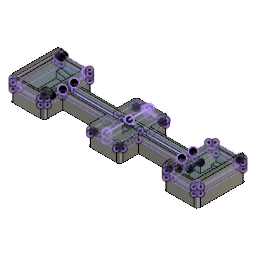
Sonaptic (Autodesk Fusion 360 design; units mm, degrees)
Autodesk Fusion 360 part; units mm, degrees
sketch "Bottom_Profile1" plane through (0, 0, 0) normal (0, 0, 1) x (1, 0, 0) in component "Bottom"
  line L0 (16, -30) -> (-16, -30)
  line L1 (-20, -26) -> (-20, 26)
  line L2 (-16, 30) -> (16, 30)
  line L3 (20, 26) -> (20, -26)
  line L4 (20, -30) -> (-20, 30) construction
  line L5 (-20, -30) -> (20, 30) construction
  line L6 (-11.5, 30) -> (11.5, 30)
  line L7 (11.5, 30) -> (11.5, -24)
  line L8 (11.5, -24) -> (-11.5, -24)
  line L9 (-11.5, -24) -> (-11.5, 30)
  line L10 (0, -24) -> (0, 30) construction
  line L11 (-11.5, 28) -> (11.5, 28)
  arc A0 (-16, 30) -> (-20, 26) centre (-16, 26) ccw
  arc A1 (20, 26) -> (16, 30) centre (16, 26) ccw
  arc A2 (16, -30) -> (20, -26) centre (16, -26) ccw
  arc A3 (-20, -26) -> (-16, -30) centre (-16, -26) ccw
  circle A4 centre (-16, 26) radius 1.25
  circle A5 centre (16, 26) radius 1.25
  circle A6 centre (16, -26) radius 1.25
  circle A7 centre (-16, -26) radius 1.25
  line L12 (0, 0) -> (75, 0) construction
  line L13 (111, -30) -> (77, -30)
  line L14 (73, -26) -> (73, 26)
  line L15 (77, 30) -> (111, 30)
  line L16 (115, 26) -> (115, -26)
  line L17 (115, -30) -> (73, 30) construction
  line L18 (73, -30) -> (115, 30) construction
  arc A8 (77, 30) -> (73, 26) centre (77, 26) ccw
  arc A9 (115, 26) -> (111, 30) centre (111, 26) ccw
  arc A10 (111, -30) -> (115, -26) centre (111, -26) ccw
  arc A11 (73, -26) -> (77, -30) centre (77, -26) ccw
  line L19 (20, 7) -> (73, 7)
  line L20 (20, -7) -> (73, -7)
  line L21 (-73, -30) -> (-115, 30) construction
  line L22 (-73, -26) -> (-73, 26)
  line L23 (-111, -30) -> (-77, -30)
  line L24 (-115, 26) -> (-115, -26)
  arc A12 (-111, 30) -> (-115, 26) centre (-111, 26) ccw
  line L25 (-115, -30) -> (-73, 30) construction
  arc A13 (-73, 26) -> (-77, 30) centre (-77, 26) ccw
  arc A14 (-77, -30) -> (-73, -26) centre (-77, -26) ccw
  arc A15 (-115, -26) -> (-111, -30) centre (-111, -26) ccw
  line L26 (-77, 30) -> (-111, 30)
  line L27 (-20, -7) -> (-73, -7)
  line L28 (-20, 7) -> (-73, 7)
  line L29 (0, 0) -> (-75, 0) construction
  circle A16 centre (-16, 26) radius 2
  circle A17 centre (16, 26) radius 2
  circle A18 centre (16, -26) radius 2
  circle A19 centre (-16, -26) radius 2
  line L30 (-73, 3.5) -> (73, 3.5)
  line L31 (73, 3.5) -> (73, -3.5)
  line L32 (73, -3.5) -> (-73, -3.5)
  line L33 (-73, -3.5) -> (-73, 3.5)
  line L34 (108, -26) -> (82, -26)
  line L35 (82, -26) -> (82, 26)
  line L36 (82, 26) -> (108, 26)
  line L37 (108, 26) -> (108, -26)
  line L38 (108, -26) -> (82, 26) construction
  line L39 (82, -26) -> (108, 26) construction
  line L40 (-82, 26) -> (-108, 26)
  line L41 (-82, -26) -> (-82, 26)
  line L42 (-108, -26) -> (-82, 26) construction
  line L43 (-82, -26) -> (-108, 26) construction
  line L44 (-108, 26) -> (-108, -26)
  line L45 (-108, -26) -> (-82, -26)
  line L46 (73, 3.5) -> (82, 3.5)
  line L47 (73, -3.5) -> (82, -3.5)
  line L48 (-73, 3.5) -> (-82, 3.5)
  line L49 (-73, -3.5) -> (-82, -3.5)
  line L50 (82, 7) -> (75, 7)
  line L51 (82, -7) -> (75, -7)
  line L52 (75, 7) -> (75, -7)
  line L53 (-82, 7) -> (-75, 7)
  line L54 (-75, 7) -> (-75, -7)
  line L55 (-82, -7) -> (-75, -7)
  line L56 (82, -20) -> (108, -20)
  line L57 (95, 0) -> (108, 0) construction
  line L58 (82, 20) -> (108, 20)
  line L59 (-82, 20) -> (-108, 20)
  line L60 (-82, -20) -> (-108, -20)
  circle A20 centre (-5.75, 26) radius 1.25
  circle A21 centre (5.75, 26) radius 1.25
  circle A22 centre (-5.75, -21) radius 1.25
  circle A23 centre (5.75, -21) radius 1.25
  circle A24 centre (-5.75, 26) radius 2
  circle A25 centre (5.75, 26) radius 2
  circle A26 centre (-5.75, -21) radius 2
  circle A27 centre (5.75, -21) radius 2
  circle A28 centre (111, 26) radius 1.25
  circle A29 centre (111, 26) radius 2
  circle A30 centre (77, -26) radius 2
  circle A31 centre (77, -26) radius 1.25
  circle A32 centre (-111, 26) radius 1.25
  circle A33 centre (-111, 26) radius 2
  circle A34 centre (-77, -26) radius 2
  circle A35 centre (-77, -26) radius 1.25
  point P0 (92.9265, 0)
  point P1 (-92.9265, 0)
  point P2 (92.9265, 0)
  point P3 (95, 0)
  point P4 (94, 0)
  point P5 (95, -23)
  point P6 (95, 23)
  point P7 (-95, 23)
  point P8 (-95, -23)
  dimension "d1" = 40
  dimension "d2" = 60
  dimension "d3" = 23
  dimension "d4" = 54
  dimension "d5" = 2
  dimension "d6" = 4
  dimension "d7" = 2.5
  dimension "d8" = 75
  dimension "d9" = 42
  dimension "d10" = 4
  dimension "d11" = 60
  dimension "d12" = 14
  dimension "d15" = 4
  dimension "d16" = 7
  dimension "d17" = 26
  dimension "d18" = 52
  dimension "d19" = 2
  dimension "d22" = 9
  dimension "d23" = 7
  dimension "d24" = 14
  dimension "d29" = 3
  dimension "d30" = 3
  dimension "d31" = 11.5
  dimension "d32" = 2.5
  dimension "d36" = 2
  dimension "d37" = 11.5
  dimension "d38" = 3
  dimension "d39" = 4
  dimension "d46" = 2.5
  dimension "d47" = 4
  constraint horizontal L0
  constraint perpendicular L0 L1
  constraint parallel L0 L2
  constraint parallel L1 L3
  constraint coincident L4 L12.start
  constraint coincident L5 L12.start
  constraint coincident L12.start L29.start
  constraint horizontal L6
  constraint vertical L7
  constraint horizontal L8
  constraint vertical L9
  constraint coincident L2 L6.start
  constraint midpoint L8 L10.start
  constraint midpoint L6 L10.end
  constraint coincident L12.start L10
  constraint coincident L9 L11.start
  constraint coincident L7 L11.end
  constraint perpendicular L7 L11
  constraint coincident L4.end L1
  constraint coincident L4.end L2
  constraint tangent L1 A0
  constraint tangent L2 A0
  constraint coincident L5.end L2
  constraint coincident L5.end L3
  constraint tangent L2 A1
  constraint tangent L3 A1
  constraint equal A0 A1
  constraint coincident L4.start L3
  constraint coincident L4.start L0
  constraint tangent L3 A2
  constraint tangent L0 A2
  constraint equal A0 A2
  constraint coincident L5.start L0
  constraint coincident L5.start L1
  constraint tangent L0 A3
  constraint tangent L1 A3
  constraint equal A0 A3
  constraint concentric A0 A4
  constraint concentric A1 A5
  constraint equal A4 A5
  constraint concentric A2 A6
  constraint concentric A3 A7
  constraint equal A4 A6
  constraint equal A4 A7
  constraint perpendicular L10 L12
  constraint horizontal L13
  constraint perpendicular L13 L14
  constraint parallel L13 L15
  constraint parallel L14 L16
  constraint horizontal L12.end P2
  constraint coincident L17.end L14
  constraint coincident L17.end L15
  constraint tangent L14 A8
  constraint tangent L15 A8
  constraint coincident L18.end L15
  constraint coincident L18.end L16
  constraint tangent L15 A9
  constraint tangent L16 A9
  constraint equal A8 A9
  constraint coincident L17.start L16
  constraint coincident L17.start L13
  constraint tangent L16 A10
  constraint tangent L13 A10
  constraint equal A8 A10
  constraint coincident L18.start L13
  constraint coincident L18.start L14
  constraint tangent L13 A11
  constraint tangent L14 A11
  constraint equal A8 A11
  constraint coincident L3 L19.start
  constraint coincident L14 L19.end
  constraint perpendicular L14 L19
  constraint symmetric L12 L19.start L20.start
  constraint symmetric L12 L19.end L20.end
  constraint symmetric L10 L12.start L29.start
  constraint symmetric L10 L12.end L29.end
  constraint symmetric L10 L17.start L25.start
  constraint symmetric L10 L18.start L21.start
  constraint symmetric L10 L17.end L25.end
  constraint symmetric L10 L18.end L21.end
  constraint symmetric L10 P2 P1
  constraint symmetric L10 L14.end L22.end
  constraint symmetric L10 L15.start A13.end
  constraint symmetric L10 A8 A13
  constraint symmetric L10 L15.end A12.start
  constraint symmetric L10 L16.start L24.start
  constraint symmetric L10 A9 A12
  constraint symmetric L10 L16.end L24.end
  constraint symmetric L10 L13.start L23.start
  constraint symmetric L10 A10 A15
  constraint symmetric L10 L13.end L23.end
  constraint symmetric L10 L14.start L22.start
  constraint symmetric L10 A11 A14
  constraint symmetric L10 L19.start L28.start
  constraint symmetric L10 L19.end L28.end
  constraint symmetric L10 L20.start L27.start
  constraint symmetric L10 L20.end L27.end
  constraint concentric A0 A16
  constraint concentric A5 A17
  constraint concentric A6 A18
  constraint concentric A7 A19
  constraint equal A16 A17
  constraint equal A16 A18
  constraint equal A16 A19
  constraint horizontal L30
  constraint vertical L31
  constraint horizontal L32
  constraint vertical L33
  constraint coincident L14 L31.end
  constraint coincident L22 L30.start
  constraint symmetric L12 L30 L32
  constraint horizontal L34
  constraint perpendicular L34 L35
  constraint parallel L34 L36
  constraint parallel L35 L37
  constraint coincident P2 P0
  constraint symmetric L10 L34.start L42.start
  constraint symmetric L10 L34.end L41.start
  constraint symmetric L10 L35.end L40.start
  constraint symmetric L10 L36.end L40.end
  constraint coincident L35 L46.end
  constraint perpendicular L35 L46
  constraint coincident L35 L47.end
  constraint perpendicular L35 L47
  constraint symmetric L10 L30.end L30.start
  constraint symmetric L10 L31.end L32.end
  constraint symmetric L10 L46.end L48.end
  constraint symmetric L10 L47.end L49.end
  constraint midpoint L38 P3
  constraint horizontal P2 P3
  constraint coincident L35 L50.start
  constraint perpendicular L35 L50
  constraint symmetric L12 L50.start L51.start
  constraint symmetric L12 L50.end L51.end
  constraint symmetric L10 L50.start L53.start
  constraint symmetric L10 L50.end L53.end
  constraint symmetric L10 L51.start L55.start
  constraint symmetric L10 L51.end L54.end
  constraint midpoint L17 P4
  constraint horizontal P2 P4
  constraint coincident L35 L56.start
  constraint coincident L37 L56.end
  constraint perpendicular L37 L56
  constraint coincident P3 L57.start
  constraint midpoint L37 L57.end
  constraint symmetric P5 L57 P6
  constraint symmetric L56.start L57 L58.start
  constraint symmetric L56.end L57 L58.end
  constraint symmetric L10 P5 P8
  constraint symmetric L10 L56.start L60.start
  constraint symmetric L10 L56.end L60.end
  constraint symmetric L10 P6 P7
  constraint symmetric L10 L58.start L59.start
  constraint symmetric L10 L58.end L59.end
  constraint symmetric L10 A20 A21
  constraint symmetric L10 A22 A23
  constraint equal A20 A22
  constraint concentric A20 A24
  constraint symmetric L10 A24 A25
  constraint concentric A22 A26
  constraint equal A24 A26
  constraint symmetric L10 A26 A27
  constraint concentric A9 A28
  constraint concentric A9 A29
  constraint concentric A11 A30
  constraint concentric A11 A31
  constraint equal A28 A31
  constraint equal A29 A30
  constraint symmetric L10 A28 A32
  constraint symmetric L10 A29 A33
  constraint symmetric L10 A30 A34
  constraint symmetric L10 A31 A35
  measures "d1" distance of L4.end L5.end
  measures "d2" distance of L5.start L4.end
  measures "d3" distance of L6.start L6.end
  measures "d4" distance of L6.start L8.end
  measures "d5" distance of L6 L11
  measures "d6" radius of A0
  measures "d7" diameter of A4
  measures "d8" distance of L12.start L12.end
  measures "d9" distance of L17.end L18.end
  measures "d10" radius of A8
  measures "d11" distance of L13 L15
  measures "d12" distance of L19 L20
  measures "d15" diameter of A16
  measures "d16" distance of L30 L32
  measures "d17" distance of L35.end L36.end
  measures "d18" distance of L34.end L35.end
  measures "d19" distance of L12.end L14
  measures "d22" distance of L14 L35
  measures "d23" distance of L50.start L50.end
  measures "d24" distance of L50 L51
  measures "d29" distance of L34 P5
  measures "d30" distance of P5 L56
  measures "d31" distance of A20.centre A21.centre
  measures "d32" diameter of A20
  measures "d36" distance of L11 A20.centre
  measures "d37" distance of A22.centre A23.centre
  measures "d38" distance of L8 A23.centre
  measures "d39" diameter of A24
  measures "d46" diameter of A28
  measures "d47" diameter of A29
extrude "Extrude2" add sketch "Bottom_Profile1" along normal blind 15 contours L0 L1 L3 L7 L8 L9 A2 A3 L32 | L3 L14 L20 L32 | L1 L22 L27 L32 | L13 L14 L15 L16 A8 A9 A10 A11 L34 L35 L36 L37 L46 L47 L50 L51 L52 | L22 L23 L24 A12 A13 A14 A15 L26 L40 L41 L44 L45 L48 L49 L53 L54 L55 | L2 L3 L7 A1 L30 | L3 L14 L19 L30 | L1 L22 L28 L30 | L1 L2 L9 A0 L30 | A16 | A17 | A18 | A19 | A29 | A30 | A33 | A34 makes body 1 in component "Bottom"
extrude "Extrude3" add sketch "Bottom_Profile1" along normal blind 3 contours L3 L7 L30 L32 | L3 L14 L30 L31 L32 | L1 L22 L30 L32 L33 | L1 L9 L30 L32 | L14 L31 L46 L47 L52 | L7 L9 L30 L32 | L22 L33 L48 L49 L54 | L35 L46 L47 L52 | L35 L47 L51 L52 | L41 L49 L54 L55 | L41 L48 L49 L54 | L35 L46 L50 L52 | L35 L37 L56 L58 | L41 L48 L53 L54 | L41 L44 L59 L60 bodies 1 in component "Bottom"
extrude "Extrude4" add sketch "Bottom_Profile1" along normal blind 5 contours L7 L8 L9 L32 | A25 | A24 | L7 L9 L11 L30 | A26 | A27 bodies 1 in component "Bottom"
extrude "Extrude5" add sketch "Bottom_Profile1" along normal up to surface (6 mm away) contours L2 L6 L7 L9 L11 bodies 1 in component "Bottom"
extrude "Extrude6" add sketch "Bottom_Profile1" along normal blind 16 contours L34 L35 L37 L56 | L41 L44 L45 L60 | L35 L36 L37 L58 | L40 L41 L44 L59 bodies 1 in component "Bottom"
sketch "Slice_Profile1" plane through (0, 0, 0) normal (0, 1, 0) x (1, 0, 0) in component "Bottom"
  line L0 (82, -3) -> (82, -6) construction
  line L1 (82, -6) -> (82, -16)
  line L2 (108, -3) -> (108, -16) construction
  line L3 (82, -6) -> (108, -6) construction
  line L4 (82, -6) -> (108, -10.5845)
  line L5 (108, -10.5845) -> (108, -16)
  line L6 (108, -16) -> (82, -16)
  line L7 (0, -1.75) -> (0, -22.5)
  line L8 (-108, -16) -> (-82, -16)
  line L9 (-82, -6) -> (-108, -10.5845)
  line L10 (-82, -6) -> (-82, -16)
  line L11 (-108, -10.5845) -> (-108, -16)
  point P0 (108, -3)
  point P1 (82, -3)
  point P2 (108, -16)
  dimension "d48" = 3
  dimension "d49" = 10
  constraint coincident P1 L0.start
  constraint vertical L0
  constraint parallel L0 L1
  constraint coincident P0 L2.start
  constraint coincident P2 L2.end
  constraint coincident L2 L3.end
  constraint perpendicular L2 L3
  constraint coincident L2 L4.end
  constraint perpendicular L1 L6
  constraint symmetric L0.end L7 L9.start
  constraint symmetric L1.end L7 L8.end
  constraint symmetric L4.end L7 L9.end
  constraint symmetric P2 L7 L8.start
  measures "d48" distance of P1 L0.end
  measures "d49" angle of L3 L4
extrude "Extrude7" cut sketch "Slice_Profile1" along normal up to surface (26 mm away) and the other way up to surface (26 mm away) bodies 1 in component "Bottom"
sketch "Fastener_Profile1" plane through (-1.4465, 0, -8.2037) normal (0.173648, 0, 0.984808) x (0, 1, 0) in component "Bottom"
  line L0 (-20, 81.7961) -> (-20, 108.1972)
  line L1 (-20, 108.1972) -> (-26, 108.1972)
  line L2 (-26, 108.1972) -> (-26, 81.7961)
  line L3 (-26, 81.7961) -> (-20, 81.7961)
  circle A0 centre (-23, 94.9967) radius 2.25
  circle A1 centre (-23, 94.9967) radius 2
  circle A2 centre (-23, 94.9967) radius 1.25
  line L4 (-23, 108.1972) -> (-23, 81.7961) construction
  line L5 (-20, 94.9967) -> (-26, 94.9967) construction
  point P0 (-23, 93.5567)
  point P1 (-23, 94.9967)
  dimension "d55" = 4.5
  dimension "d56" = 4
  dimension "d57" = 2.5
  constraint midpoint L1 L4.start
  constraint midpoint L3 L4.end
  constraint coincident P1 L4
  constraint coincident P1 A0.centre
  constraint midpoint L0 L5.start
  constraint midpoint L2 L5.end
  constraint coincident L4 P1
  constraint coincident L5 P1
  measures "d55" diameter of A0
  measures "d56" diameter of A1
  measures "d57" diameter of A2
sketch "Fastener_Profile2" plane through (1.4465, 0, -8.2037) normal (-0.173648, 0, 0.984808) x (0, -1, 0) in component "Bottom"
  line L0 (-20, 81.7961) -> (-20, 108.1972)
  line L1 (-20, 108.1972) -> (-26, 108.1972)
  line L2 (-26, 108.1972) -> (-26, 81.7961)
  line L3 (-26, 81.7961) -> (-20, 81.7961)
  circle A0 centre (-23, 94.9967) radius 2.25
  circle A1 centre (-23, 94.9967) radius 2
  circle A2 centre (-23, 94.9967) radius 1.25
  line L4 (-23, 108.1972) -> (-23, 81.7961) construction
  line L5 (-26, 94.9967) -> (-20, 94.9967) construction
  point P0 (-23, 93.5567)
  point P1 (-23, 94.9967)
  dimension "d58" = 4.5
  dimension "d59" = 4
  dimension "d60" = 2.5
  constraint midpoint L1 L4.start
  constraint midpoint L3 L4.end
  constraint midpoint L2 L5.start
  constraint midpoint L0 L5.end
  constraint coincident L4 P1
  constraint coincident L5 P1
  constraint coincident P1 A0.centre
  measures "d58" diameter of A0
  measures "d59" diameter of A1
  measures "d60" diameter of A2
extrude "Extrude8" cut sketch "Fastener_Profile2" against normal blind 6 contours A2 bodies 1 in component "Bottom"
extrude "Extrude9" cut sketch "Fastener_Profile2" against normal blind 5 contours A1 bodies 1 in component "Bottom"
extrude "Extrude10" cut sketch "Fastener_Profile2" against normal blind 1 contours A0 bodies 1 in component "Bottom"
extrude "Extrude11" cut sketch "Fastener_Profile1" against normal blind 6 contours A2 bodies 1 in component "Bottom"
extrude "Extrude12" cut sketch "Fastener_Profile1" against normal blind 5 contours A1 bodies 1 in component "Bottom"
extrude "Extrude13" cut sketch "Fastener_Profile1" against normal blind 1 contours A0 bodies 1 in component "Bottom"
extrude "Extrude14" cut sketch "Bottom_Profile1" along normal blind 5 contours A16 | A17 | A18 | A19 | A29 | A30 | A33 | A34 bodies 1 in component "Bottom"
extrude "Extrude15" cut sketch "Bottom_Profile1" along normal blind 3 contours A25 | A24 | A26 | A27 bodies 1 in component "Bottom"
sketch "Top_Profile" plane through (0, 0, 15) normal (0, 0, 1) x (-1, 0, 0) in component "Top"
  circle A0 centre (111, -26) radius 1.25
  circle A1 centre (77, 26) radius 1.25
  circle A2 centre (-111, -26) radius 1.25
  circle A3 centre (16, 26) radius 1.25
  circle A4 centre (-16, 26) radius 1.25
  circle A5 centre (16, -26) radius 1.25
  circle A6 centre (-77, 26) radius 1.25
  circle A7 centre (-16, -26) radius 1.25
  line L0 (82, -7) -> (75, -7)
  line L1 (75, -7) -> (75, -3.5)
  line L2 (75, -3.5) -> (11.5, -3.5)
  line L3 (11.5, -3.5) -> (11.5, -30)
  line L4 (11.5, -30) -> (16, -30)
  arc A8 (16, -30) -> (20, -26) centre (16, -26) ccw
  line L5 (20, -26) -> (20, -7)
  line L6 (20, -7) -> (73, -7)
  line L7 (73, -7) -> (73, -26)
  arc A9 (73, -26) -> (77, -30) centre (77, -26) ccw
  line L8 (77, -30) -> (111, -30)
  arc A10 (111, -30) -> (115, -26) centre (111, -26) ccw
  line L9 (115, -26) -> (115, 26)
  arc A11 (115, 26) -> (111, 30) centre (111, 26) ccw
  line L10 (111, 30) -> (77, 30)
  arc A12 (77, 30) -> (73, 26) centre (77, 26) ccw
  line L11 (73, 26) -> (73, 7)
  line L12 (73, 7) -> (20, 7)
  line L13 (20, 7) -> (20, 26)
  arc A13 (20, 26) -> (16, 30) centre (16, 26) ccw
  line L14 (16, 30) -> (-16, 30)
  arc A14 (-16, 30) -> (-20, 26) centre (-16, 26) ccw
  line L15 (-20, 26) -> (-20, 7)
  line L16 (-20, 7) -> (-73, 7)
  line L17 (-73, 7) -> (-73, 26)
  arc A15 (-73, 26) -> (-77, 30) centre (-77, 26) ccw
  line L18 (-77, 30) -> (-111, 30)
  arc A16 (-111, 30) -> (-115, 26) centre (-111, 26) ccw
  line L19 (-115, 26) -> (-115, -26)
  arc A17 (-115, -26) -> (-111, -30) centre (-111, -26) ccw
  line L20 (-111, -30) -> (-77, -30)
  arc A18 (-77, -30) -> (-73, -26) centre (-77, -26) ccw
  line L21 (-73, -26) -> (-73, -7)
  line L22 (-73, -7) -> (-20, -7)
  line L23 (-20, -7) -> (-20, -26)
  arc A19 (-20, -26) -> (-16, -30) centre (-16, -26) ccw
  line L24 (-16, -30) -> (-11.5, -30)
  line L25 (-11.5, -30) -> (-11.5, -3.5)
  line L26 (-11.5, -3.5) -> (-75, -3.5)
  line L27 (-75, -3.5) -> (-75, -7)
  line L28 (-75, -7) -> (-82, -7)
  line L29 (-82, -7) -> (-82, -26)
  line L30 (-82, -26) -> (-108, -26)
  line L31 (-108, -26) -> (-108, 26)
  line L32 (-108, 26) -> (-82, 26)
  line L33 (-82, 26) -> (-82, 7)
  line L34 (-82, 7) -> (-75, 7)
  line L35 (-75, 7) -> (-75, 3.5)
  line L36 (-75, 3.5) -> (-11.5, 3.5)
  line L37 (-11.5, 3.5) -> (-11.5, 24)
  line L38 (-11.5, 24) -> (11.5, 24)
  line L39 (11.5, 24) -> (11.5, 3.5)
  line L40 (11.5, 3.5) -> (75, 3.5)
  line L41 (75, 3.5) -> (75, 7)
  line L42 (75, 7) -> (82, 7)
  line L43 (82, 7) -> (82, 26)
  line L44 (82, 26) -> (108, 26)
  line L45 (108, 26) -> (108, -26)
  line L46 (108, -26) -> (82, -26)
  line L47 (82, -26) -> (82, -7)
  line L48 (16, -30) -> (-16, -30)
  line L49 (11.5, -28) -> (-11.5, -28)
  line L50 (-11.5, -30) -> (11.5, -30)
  line L51 (11.5, -30) -> (11.5, -28)
  line L52 (11.5, -28) -> (-11.5, -28)
  line L53 (-11.5, -28) -> (-11.5, -30)
  circle A20 centre (16, 26) radius 2
  circle A21 centre (16, 26) radius 2.25
  circle A22 centre (-16, 26) radius 2
  circle A23 centre (-16, 26) radius 2.25
  circle A24 centre (-16, -26) radius 2
  circle A25 centre (16, -26) radius 2
  circle A26 centre (16, -26) radius 2.25
  circle A27 centre (-16, -26) radius 2.25
  line L54 (-82, 7) -> (-82, -7)
  line L55 (82, 7) -> (82, -7)
  dimension "d87" = 4
  dimension "d88" = 4.5
  constraint concentric A3 A20
  constraint concentric A3 A21
  constraint concentric A4 A22
  constraint concentric A22 A23
  constraint concentric A7 A24
  constraint concentric A5 A25
  constraint concentric A25 A26
  constraint concentric A24 A27
  constraint equal A21 A27
  constraint equal A21 A23
  constraint equal A21 A26
  constraint equal A20 A25
  constraint equal A20 A24
  constraint equal A20 A22
  constraint coincident L33.end L34.start
  constraint coincident L28.end L29.start
  constraint coincident L42.end L43.start
  constraint coincident L0.start L47.end
  measures "d87" diameter of A20
  measures "d88" diameter of A21
extrude "Extrude1" add sketch "Top_Profile" along normal blind 7 separate body contours A3 | A4 | A5 | A7 | L0 L1 L2 L3 L4 A8 L5 L6 L7 A9 L8 A10 L9 A11 L10 A12 L11 L12 L13 A13 L14 A14 L15 L16 L17 A15 L18 A16 L19 A17 L20 A18 L21 L22 L23 A19 L24 L25 L26 L27 L28 L29 L30 L31 L32 L33 L34 L35 L36 L37 L38 L39 L40 L41 L42 L43 L44 L45 L46 L47 L48 L51 L53 | L0 L1 L2 L3 L25 L26 L27 L28 L34 L35 L36 L37 L38 L39 L40 L41 L42 L49 L52 L54 L55 | L3 L25 L48 L49 L50 L51 L52 L53 | A20 | A21 | A22 | A23 | A24 | A25 | A26 | A27 makes body 2 in component "Top"
extrude "Extrude2'" add sketch "Top_Profile" against normal blind 3 contours L3 L25 L48 L49 L50 L51 L52 L53 bodies 2 in component "Top"
extrude "Extrude4'" cut sketch "Top_Profile" along normal blind 3 contours L43 L44 L45 L46 L47 L55 | L0 L1 L2 L3 L25 L26 L27 L28 L34 L35 L36 L37 L38 L39 L40 L41 L42 L49 L52 L54 L55 | L29 L30 L31 L32 L33 L54 bodies 2 in component "Top"
extrude "Extrude5'" cut sketch "Top_Profile" along normal blind 6 contours A3 | A4 | A5 | A7 bodies 2 in component "Top"
extrude "Extrude6'" cut sketch "Top_Profile" along normal blind 5 contours A20 | A22 | A24 | A25 bodies 2 in component "Top"
extrude "Extrude7'" cut sketch "Top_Profile" along normal blind 1 contours A21 | A23 | A26 | A27 bodies 2 in component "Top"
sketch "Side_Profile" plane through (0, 0, 0) normal (1, 0, 0) x (0, 1, 0) in component "Strip"
  line L0 (-26, 15) -> (26, 15)
  line L1 (-26, 22) -> (26, 22)
  circle A0 centre (0, 17.75) radius 6.25
  line L2 (6.25, 11.5) -> (-6.25, 11.5) construction
  line L3 (-6.25, 11.5) -> (-6.25, 24)
  line L4 (-6.25, 24) -> (6.25, 24) construction
  line L5 (6.25, 24) -> (6.25, 11.5)
  line L6 (6.25, 11.5) -> (-6.25, 24) construction
  line L7 (-6.25, 11.5) -> (6.25, 24) construction
  point P0 (0, 22)
  point P1 (0, 17.75)
  dimension "d81" = 12.5
  dimension "d82" = 2
  constraint vertical origin P1
  constraint midpoint L1 P0
  constraint horizontal L2
  constraint perpendicular L2 L3
  constraint parallel L2 L4
  constraint parallel L3 L5
  constraint coincident L6 P1
  constraint coincident L7 P1
  constraint coincident P1 A0.centre
  constraint tangent A0 L4
  constraint tangent A0 L5
  measures "d81" diameter of A0
  measures "d82" distance of P0 L4
sketch "Profile_Bottom" plane through (0, 0, 22) normal (0, 0, 1) x (-1, 0, 0) in component "Cover"
  line L0 (-82, 26) -> (-82, -26)
  line L1 (-82, -26) -> (-108, -26)
  line L2 (-108, -26) -> (-108, 26)
  line L3 (-108, 26) -> (-82, 26)
  circle A0 centre (-77, 26) radius 1.25
  circle A1 centre (-111, -26) radius 1.25
  circle A2 centre (111, -26) radius 1.25
  circle A3 centre (77, 26) radius 1.25
  line L4 (82, -26) -> (82, 26)
  line L5 (82, 26) -> (108, 26)
  line L6 (108, 26) -> (108, -26)
  line L7 (108, -26) -> (82, -26)
  arc A4 (16, -30) -> (20, -26) centre (16, -26) ccw
  line L8 (20, -26) -> (20, -7)
  line L9 (20, -7) -> (73, -7)
  line L10 (73, -7) -> (73, -26)
  arc A5 (73, -26) -> (77, -30) centre (77, -26) ccw
  line L11 (77, -30) -> (111, -30)
  arc A6 (111, -30) -> (115, -26) centre (111, -26) ccw
  line L12 (115, -26) -> (115, 26)
  arc A7 (115, 26) -> (111, 30) centre (111, 26) ccw
  line L13 (111, 30) -> (77, 30)
  arc A8 (77, 30) -> (73, 26) centre (77, 26) ccw
  line L14 (73, 26) -> (73, 7)
  line L15 (73, 7) -> (20, 7)
  line L16 (20, 7) -> (20, 26)
  arc A9 (20, 26) -> (16, 30) centre (16, 26) ccw
  line L17 (16, 30) -> (-16, 30)
  arc A10 (-16, 30) -> (-20, 26) centre (-16, 26) ccw
  line L18 (-20, 26) -> (-20, 7)
  line L19 (-20, 7) -> (-73, 7)
  line L20 (-73, 7) -> (-73, 26)
  arc A11 (-73, 26) -> (-77, 30) centre (-77, 26) ccw
  line L21 (-77, 30) -> (-111, 30)
  arc A12 (-111, 30) -> (-115, 26) centre (-111, 26) ccw
  line L22 (-115, 26) -> (-115, -26)
  arc A13 (-115, -26) -> (-111, -30) centre (-111, -26) ccw
  line L23 (-111, -30) -> (-77, -30)
  arc A14 (-77, -30) -> (-73, -26) centre (-77, -26) ccw
  line L24 (-73, -26) -> (-73, -7)
  line L25 (-73, -7) -> (-20, -7)
  line L26 (-20, -7) -> (-20, -26)
  arc A15 (-20, -26) -> (-16, -30) centre (-16, -26) ccw
  line L27 (-16, -30) -> (16, -30)
  line L28 (73, -7) -> (73, 7)
  line L29 (-73, -7) -> (-73, 7)
  arc A16 (-77, -30) -> (-73, -26) centre (-77, -26) ccw
  line L30 (-111, -30) -> (-77, -30)
  line L31 (-73, -26) -> (-73, -7)
  line L32 (-73, 7) -> (-73, 26)
  line L33 (73, 26) -> (73, 7)
  line L34 (73, -7) -> (73, -26)
  arc A17 (73, -26) -> (77, -30) centre (77, -26) ccw
  arc A18 (77, 30) -> (73, 26) centre (77, 26) ccw
  circle A19 centre (77, 26) radius 1.25
  arc A20 (111, -30) -> (115, -26) centre (111, -26) ccw
  line L35 (77, -30) -> (111, -30)
  line L36 (115, -26) -> (115, 26)
  arc A21 (115, 26) -> (111, 30) centre (111, 26) ccw
  line L37 (111, 30) -> (77, 30)
  circle A22 centre (111, -26) radius 1.25
  arc A23 (-73, 26) -> (-77, 30) centre (-77, 26) ccw
  circle A24 centre (-77, 26) radius 1.25
  arc A25 (-115, -26) -> (-111, -30) centre (-111, -26) ccw
  circle A26 centre (-111, -26) radius 1.25
  line L38 (-77, 30) -> (-111, 30)
  arc A27 (-111, 30) -> (-115, 26) centre (-111, 26) ccw
  line L39 (-115, 26) -> (-115, -26)
  circle A28 centre (-111, -26) radius 2.25
  circle A29 centre (-111, -26) radius 1.9
  circle A30 centre (-77, 26) radius 2.25
  circle A31 centre (-77, 26) radius 1.9
  circle A32 centre (111, -26) radius 2.25
  circle A33 centre (111, -26) radius 1.9
  circle A34 centre (77, 26) radius 2.25
  circle A35 centre (77, 26) radius 1.9
  line L40 (108, -26) -> (108, -30)
  line L41 (82, 20) -> (73, 20)
  line L42 (0, -1.75) -> (0, -22.5)
  line L43 (-108, -26) -> (-108, -30)
  line L44 (-82, 20) -> (-73, 20)
  point P0 (-111, 26)
  point P1 (82, 20)
  dimension "d123" = 4.5
  dimension "d124" = 3.8
  dimension "d125" = 4.5
  dimension "d126" = 3.8
  constraint coincident L9.end L10.start
  constraint coincident L14.end L15.start
  constraint coincident L24.end L25.start
  constraint coincident L19.end L20.start
  constraint concentric A26 A28
  constraint concentric A25 A29
  constraint concentric A24 A30
  constraint concentric A23 A31
  constraint equal A29 A31
  constraint equal A28 A30
  constraint concentric A20 A32
  constraint concentric A22 A33
  constraint concentric A18 A34
  constraint concentric A19 A35
  constraint equal A33 A35
  constraint equal A32 A34
  constraint coincident L6.end L7.start
  constraint coincident L35 L40.end
  constraint perpendicular L35 L40
  constraint coincident P1 L41.start
  constraint coincident L14 L41.end
  constraint perpendicular L14 L41
  constraint symmetric L6.end L42 L1.end
  constraint symmetric L40.end L42 L43.end
  constraint symmetric P1 L42 L44.start
  constraint symmetric L41.end L42 L44.end
  measures "d123" diameter of A28
  measures "d124" diameter of A29
  measures "d125" diameter of A32
  measures "d126" diameter of A33
extrude "Extrude11'" add sketch "Profile_Bottom" along normal blind 6 separate body contours L0 L2 L3 L20 A11 L21 A12 L22 A13 L23 L30 L32 A23 A25 L38 A27 L39 L43 L44 | L4 L5 L6 L11 A6 L12 A7 L13 A8 L14 L33 A18 A20 L35 L36 A21 L37 L40 L41 | A0 A24 | A1 A26 | A2 A22 | A3 A19 | A28 | A29 | A30 | A31 | A32 | A33 | A34 | A35 makes body 3 at (-110.3333, 10, 22) makes body 4 at (110.3333, 10, 22) in component "Cover"
chamfer "Chamfer3" distance 2 angle 45 6 edges at (82, -23, 28) (95, -26, 28) (108, 2, 28) (-108, 2, 28) (-95, -26, 28) (-82, -23, 28) on bodies 3 4 in component "Cover"
extrude "Extrude12'" cut sketch "Profile_Bottom" along normal blind 5 contours A0 A24 | A1 A26 | A2 A22 | A3 A19 | A29 | A31 | A33 | A35 bodies 3 4 in component "Cover"
extrude "Extrude13'" cut sketch "Profile_Bottom" along normal blind 1 contours A28 | A30 | A32 | A34 bodies 3 4 in component "Cover"
extrude "Extrude17" cut sketch "Side_Profile" along normal mid plane 151 contours L0 L1 A0 | L0 A0 | L1 A0 bodies 1 in component "Bottom"
extrude "Extrude9'" cut sketch "Side_Profile" along normal mid plane 151 contours L0 L1 A0 | L0 A0 | L1 A0 bodies 2 in component "Top"
component "Bottom" placed x (1, 0, 0) y (0, 1, 0) z (0, 0, 1) at (0, 0, 0)
component "Top" placed x (1, 0, 0) y (0, 1, 0) z (0, 0, 1) at (0, 0, 0)
component "Strip" placed x (1, 0, 0) y (0, 1, 0) z (0, 0, 1) at (0, 0, 0)
component "Cover" placed x (1, 0, 0) y (0, 1, 0) z (0, 0, 1) at (0, 0, 0)
equation "d22 = 7 mm + 2 mm"
equation "d49 = tilt_deg"
equation "tilt_deg = 10 deg"
